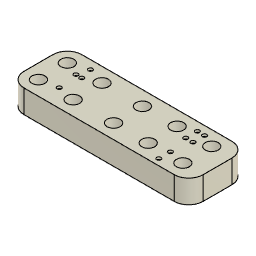
M3 Heat Set Insert Practice Block (Autodesk Fusion 360 design; units mm, degrees)
Autodesk Fusion 360 part; units mm, degrees
sketch "Sketch1" plane through (0, 0, 0) normal (0, 0, 1) x (1, 0, 0)
  circle A0 centre (-13, 0.815) radius 2.25
  circle A1 centre (-1, 0.815) radius 2.25
  circle A2 centre (13, 0.815) radius 2.25
  circle A3 centre (25, 0.815) radius 2.25
  circle A4 centre (37, 0.815) radius 2.25
  line L0 (-13, 0.815) -> (37, 0.815) construction
  circle A5 centre (-13, 10.815) radius 2.25
  circle A6 centre (-1, 10.815) radius 2.25
  circle A7 centre (13, 10.815) radius 2.25
  circle A8 centre (25, 10.815) radius 2.25
  circle A9 centre (37, 10.815) radius 2.25
  line L1 (-3, 4) -> (29, 4) construction
  line L2 (35.0527, 5.815) -> (-9.0686, 5.815) construction
  line L3 (-13, 10.815) -> (37, 10.815) construction
  line L4 (-13, 0.815) -> (37, 0.815) construction
  line L5 (-13, 0.815) -> (-13, 5.815) construction
  line L6 (-13, 5.815) -> (-13, 10.815) construction
  line L7 (-13, 5.815) -> (30, 5.815)
  line L8 (-13, 5.815) -> (-13, 15.815) construction
  line L9 (-13, 15.815) -> (39, 15.815)
  line L10 (-13, -4.185) -> (39, -4.185)
  line L11 (-13, 10.815) -> (-18, 10.815) construction
  arc A10 (-13, 15.815) -> (-18, 10.815) centre (-13, 10.815) ccw
  arc A11 (-18, 0.815) -> (-13, -4.185) centre (-13, 0.815) ccw
  line L12 (-18, 10.815) -> (-18, 0.815)
  line L13 (13, -4.185) -> (13, 15.815) construction
  arc A12 (44, 10.815) -> (39, 15.815) centre (39, 10.815) ccw
  line L14 (44, 10.815) -> (44, 0.815)
  arc A13 (39, -4.185) -> (44, 0.815) centre (39, 0.815) ccw
  point P0 (13, 4)
  dimension "d6" = 4.5
  dimension "d7" = 4.5
  dimension "d8" = 4.5
  dimension "d9" = 4.5
  dimension "d10" = 4.5
  dimension "d29" = 4.5
  dimension "d30" = 4.5
  dimension "d31" = 4.5
  dimension "d32" = 4.5
  dimension "d33" = 4.5
  dimension "d38" = 5
  dimension "d39" = 5
  dimension "d41" = 10
  dimension "M3_insert_taper_Ref" = -4
  constraint coincident A0.centre L0.start
  constraint coincident A4.centre L0.end
  constraint midpoint L1 P0
  constraint coincident A5.centre L3.start
  constraint coincident A9.centre L3.end
  constraint horizontal L3
  constraint coincident A8.centre L3
  constraint coincident A7.centre L3
  constraint coincident A6.centre L3
  constraint coincident A3.centre L4
  constraint coincident A2.centre L0
  constraint coincident A1.centre L0
  constraint perpendicular L1 L5
  constraint perpendicular L4 L5
  constraint perpendicular L3 L6
  constraint coincident L2 L5.end
  constraint coincident L2 L7.end
  constraint perpendicular L5 L7
  constraint perpendicular L7 L8
  constraint perpendicular L8 L9
  constraint symmetric L2 L8.end L10.start
  constraint symmetric L2 L9.end L10.end
  constraint perpendicular L8 L11
  constraint tangent L9 A10
  constraint symmetric L2 L11.end A11.start
  constraint symmetric L2 A10 A11
  constraint tangent A11 L12
  constraint midpoint L10 L13.start
  constraint midpoint L9 L13.end
  constraint symmetric L8.end L13 L9.end
  constraint symmetric L11.end L13 A12.start
  constraint symmetric A10 L13 A12
  constraint symmetric L10.start L13 L10.end
  constraint symmetric A11.start L13 L14.end
  constraint symmetric A11 L13 A13
  measures "d6" diameter of A0
  measures "d7" diameter of A1
  measures "d8" diameter of A2
  measures "d9" diameter of A3
  measures "d10" diameter of A4
  measures "d29" diameter of A5
  measures "d30" diameter of A6
  measures "d31" diameter of A7
  measures "d32" diameter of A8
  measures "d33" diameter of A9
  measures "d38" distance of L5.end A5.centre
  measures "d39" distance of A0.centre L5.end
  measures "d41" distance of L5.end L8.end
extrude "Extrude1" add sketch "Sketch1" along normal blind 8 contours A0 | A1 | A2 | A3 | A4 | A5 | A6 | A7 | A8 | A9 | L9 L10 A10 A11 L12 A12 L14 A13
extrude "Extrude4" cut sketch "Sketch1" against normal blind 5.8 draft -4 from surface at 8 contours A0 | A1 | A2 | A3 | A4 | A5 | A6 | A7 | A8 | A9
sketch "Sketch2" plane through (0, 0, 8) normal (0, 0, 1) x (-1, 0, 0)
  line L0 (11, 0) -> (3, 0) construction
  line L1 (7, 0) -> (7, -2) construction
  circle A0 centre (7, -2) radius 0.75
  line L2 (-27.5, 0) -> (-35.5, 0) construction
  line L3 (-35.5, 0) -> (-31.5, 0) construction
  line L4 (-31.5, 0) -> (-31.5, -2) construction
  circle A1 centre (-31.5, -2) radius 0.75
  circle A2 centre (-31.5, 2) radius 0.75
  line L5 (7, -10.815) -> (7, -12.815) construction
  line L6 (7, -12.815) -> (7, -10.815) construction
  line L7 (7, -10.815) -> (7, -8.815) construction
  line L8 (7, -8.815) -> (8, -8.815) construction
  line L9 (8, -8.815) -> (6, -8.815) construction
  circle A3 centre (8, -8.815) radius 0.75
  circle A4 centre (6, -8.815) radius 0.75
  circle A5 centre (7, -12.815) radius 0.75
  line L10 (-13, -10.815) -> (-13, -0.815) construction
  circle A6 centre (-32.5, -8.815) radius 0.75
  circle A7 centre (-30, -8.815) radius 0.75
  circle A8 centre (-32.5, -12.815) radius 0.75
  circle A9 centre (-30, -12.815) radius 0.75
  arc A10 (13, -15.815) -> (18, -10.815) centre (13, -10.815) ccw
  line L11 (18, -10.815) -> (18, -0.815)
  arc A11 (18, -0.815) -> (13, 4.185) centre (13, -0.815) ccw
  line L12 (13, 4.185) -> (-39, 4.185)
  arc A12 (-39, 4.185) -> (-44, -0.815) centre (-39, -0.815) ccw
  line L13 (-44, -0.815) -> (-44, -10.815)
  arc A13 (-44, -10.815) -> (-39, -15.815) centre (-39, -10.815) ccw
  line L14 (-39, -15.815) -> (13, -15.815)
  circle A14 centre (13, -0.815) radius 2.25
  circle A15 centre (-25, -0.815) radius 2.25
  circle A16 centre (-37, -0.815) radius 2.25
  circle A17 centre (-13, -10.815) radius 2.25
  circle A18 centre (1, -0.815) radius 2.25
  circle A19 centre (13, -10.815) radius 2.25
  circle A20 centre (-25, -10.815) radius 2.25
  circle A21 centre (-37, -10.815) radius 2.25
  circle A22 centre (1, -10.815) radius 2.25
  circle A23 centre (-13, -0.815) radius 2.25
  dimension "d14" = 1.5
  dimension "d15" = 2
  dimension "d16" = 1.5
  dimension "d21" = 1.5
  dimension "d22" = 1.5
  dimension "d23" = 1.5
  dimension "d35" = 1
  dimension "d36" = 1
  constraint midpoint L0 L1.start
  constraint perpendicular L0 L1
  constraint coincident L1.end A0.centre
  constraint midpoint L2 L3.end
  constraint perpendicular L3 L4
  constraint coincident L4.end A1.centre
  constraint symmetric L3 A1 A2
  constraint perpendicular L7 L8
  constraint perpendicular L7 L9
  constraint coincident L8.end L9.start
  constraint coincident L9.end A4.centre
  constraint coincident L5.end L6.start
  measures "d14" diameter of A0
  measures "d15" distance of L3.end L4.end
  measures "d16" diameter of A1
  measures "d21" diameter of A3
  measures "d22" diameter of A4
  measures "d23" diameter of A5
  measures "d35" distance of L7.end L9.end
  measures "d36" distance of L7.end L8.end
extrude "Extrude2" cut sketch "Sketch2" against normal blind 0.8 contours A0 | A1 | A2 | A3 | A4 | A5 | A6 | A7 | A8 | A9
equation "d6 = d30"
equation "d7 = d30"
equation "d8 = d30"
equation "d9 = d30"
equation "d10 = d30"
equation "d16 = d14"
equation "d21 = d14"
equation "d22 = d14"
equation "d23 = d14"
equation "d26 = -insert_depth"
equation "d27 = taper_angle"
equation "d29 = insert_diameter"
equation "d30 = d29"
equation "d31 = d30"
equation "d32 = d30"
equation "d33 = d30"
equation "M3_insert_dia_Ref = 4.5 mm" comment "Diameter of a hole for an M3 brass insert"
equation "M3_insert_depth_Ref = 5.8 mm" comment "Standard depth of an M3 brass insert"
equation "M3_insert_taper_Ref = -4 deg" comment "Taper angle for an M3 insert hole."
equation "insert_diameter = M3_insert_dia_Ref"
equation "taper_angle = M3_insert_taper_Ref"
equation "insert_depth = M3_insert_depth_Ref"
